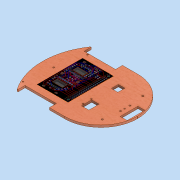
# Autodesk Inventor part: Version Raspberry Pi 3 en adelante
Saved by Autodesk Inventor 2022 (Build 260153000, 153)
## iProperties
Created: 2021-09-27
Part Number: Version Raspberry Pi 3 en adelante
Material: Madera (nogal)
Document SubType Name: Modeling
Designer: Julio R
Density: 0.55 g/cm^3
Appearance: Nogal - Natural pulido
Author: Julio R
Autodesk Inventor part; units mm, degrees
ref_plane "YZ Plane" through (0, 0, 0) normal (1, 0, 0) x (0, 1, 0)
ref_plane "XZ Plane" through (0, 0, 0) normal (0, 1, 0) x (-1, 0, 0)
ref_plane "XY Plane" through (0, 0, 0) normal (0, 0, 1) x (1, 0, 0)
sketch "Boceto2" plane through (0, 0, 0) normal (0, 1, 0) x (-1, 0, 0)
  line L0 (-78.5, 29.7) -> (-78.5, -49.3)
  line L1 (-75.5, -52.3) -> (-25.5, -52.3)
  line L2 (-22.5, -49.3) -> (-22.5, 29.7)
  line L3 (-25.5, 32.7) -> (-75.5, 32.7)
  circle A0 centre (-75, -28.8) radius 1.25
  line L4 (0, 6.809) -> (0, -6.809)
  line L5 (10.65, 0) -> (-10.65, 0) construction
  circle A1 centre (-26, -28.8) radius 1.25
  circle A2 centre (-75, 29.2) radius 1.25
  circle A3 centre (-26, 29.2) radius 1.25
  line L6 (7.5, -42.3) -> (-7, -42.3)
  line L7 (-7, -42.3) -> (-7, -25)
  line L8 (-7, -25) -> (7.5, -25)
  line L9 (7.5, -25) -> (7.5, -42.3)
  arc A4 (9.0958, -33.5419) -> (9.0958, -25.0441) centre (9, -29.293) ccw
  line L10 (9.0958, -33.5419) -> (7.5, -42.3)
  line L11 (9.0958, -25.0441) -> (7.5, -25.0441)
  arc A5 (9.5, -30.443) -> (9.5, -28.143) centre (9.5, -29.293) ccw
  line L12 (9.5, -30.443) -> (7.5, -30.443)
  line L13 (7.5, -30.443) -> (7.5, -28.143)
  line L14 (7.5, -28.143) -> (9.5, -28.143)
  line L15 (9.5, -28.143) -> (9.5, -30.443)
  arc A6 (-9.0958, -25.0441) -> (-9.0958, -33.5419) centre (-9, -29.293) ccw
  line L16 (-9.0958, -33.5419) -> (-7, -42.3)
  line L17 (-9.0958, -25.0441) -> (-7.5, -25.0441)
  arc A7 (-9.5, -28.143) -> (-9.5, -30.443) centre (-9.5, -29.293) ccw
  line L18 (-9.5, -30.443) -> (-7.5, -30.443)
  line L19 (-7.5, -30.443) -> (-7.5, -28.143)
  line L20 (-7.5, -28.143) -> (-9.5, -28.143)
  line L21 (-9.5, -28.143) -> (-9.5, -30.443)
  line L22 (7.5, 42.3) -> (-7, 42.3)
  line L23 (-7, 42.3) -> (-7, 25)
  line L24 (-7, 25) -> (7.5, 25)
  line L25 (7.5, 25) -> (7.5, 42.3)
  arc A8 (9.0958, 25.0441) -> (9.0958, 33.5419) centre (9, 29.293) ccw
  line L26 (9.0958, 33.5419) -> (7.5, 42.3)
  line L27 (9.0958, 25.0441) -> (7.5, 25.0441)
  arc A9 (9.5, 28.143) -> (9.5, 30.443) centre (9.5, 29.293) ccw
  line L28 (9.5, 30.443) -> (7.5, 30.443)
  line L29 (7.5, 30.443) -> (7.5, 28.143)
  line L30 (7.5, 28.143) -> (9.5, 28.143)
  line L31 (9.5, 28.143) -> (9.5, 30.443)
  line L32 (-9.0958, 25.0441) -> (-7.5, 25.0441)
  line L33 (-7.5, 28.143) -> (-9.5, 28.143)
  line L34 (-7.5, 30.443) -> (-7.5, 28.143)
  line L35 (-9.5, 28.143) -> (-9.5, 30.443)
  line L36 (-9.5, 30.443) -> (-7.5, 30.443)
  arc A10 (-9.5, 30.443) -> (-9.5, 28.143) centre (-9.5, 29.293) ccw
  line L37 (-9.0958, 33.5419) -> (-7, 42.3)
  arc A11 (-9.0958, 33.5419) -> (-9.0958, 25.0441) centre (-9, 29.293) ccw
  line L38 (10.3604, -4.25) -> (-9.8396, -4.25)
  line L39 (-9.8396, -4.25) -> (-9.8396, 4.25)
  line L40 (-9.8396, 4.25) -> (10.3604, 4.25)
  line L41 (10.3604, 4.25) -> (10.3604, -4.25)
  line L42 (35.3604, -42.3) -> (-82.3941, -42.3)
  line L43 (-82.3941, -42.3) -> (-82.3941, 42.3)
  line L44 (-82.3941, 42.3) -> (35.3604, 42.3)
  line L45 (35.3604, 42.3) -> (35.3604, -42.3)
  line L46 (-84.1886, -12.75) -> (-94.1886, -12.75)
  line L47 (-94.1886, -12.75) -> (-94.1886, 12.75)
  line L48 (-94.1886, 12.75) -> (-84.1886, 12.75)
  line L49 (-84.1886, 12.75) -> (-84.1886, -12.75)
  line L50 (22.5, 52.3) -> (-22.5, 52.3)
  line L51 (-22.5, 52.3) -> (-22.5, 42.3)
  line L52 (-22.5, 42.3) -> (22.5, 42.3)
  line L53 (22.5, 42.3) -> (22.5, 52.3)
  line L54 (22.5, -52.3) -> (-22.5, -52.3)
  line L55 (-22.5, -52.3) -> (-22.5, -42.3)
  line L56 (-22.5, -42.3) -> (22.5, -42.3)
  line L57 (22.5, -42.3) -> (22.5, -52.3)
  line L58 (22.5, 52.3) -> (23.5693, 52.3)
  line L59 (-22.5, 52.3) -> (-44.8693, 52.3)
  line L60 (22.5, -52.3) -> (23.5693, -52.3)
  line L61 (-22.5, -52.3) -> (-44.8693, -52.3)
  circle A12 centre (-77.6976, 5.7579) radius 1.15
  circle A13 centre (-77.6976, -7.7041) radius 1.15
  arc A14 (23.5693, -52.3) -> (23.5693, 52.3) centre (-52.609, 0) ccw
  line L62 (7.5, -18) -> (-7, -18)
  line L63 (-7, -18) -> (-7, -11.2)
  line L64 (-7, -11.2) -> (7.5, -11.2)
  line L65 (7.5, -11.2) -> (7.5, -18)
  line L66 (7.5, 11.5) -> (-7, 11.5)
  line L67 (-7, 11.5) -> (-7, 18.3)
  line L68 (-7, 18.3) -> (7.5, 18.3)
  line L69 (7.5, 18.3) -> (7.5, 11.5)
  circle A15 centre (24.1703, -0.4774) radius 1
  circle A16 centre (11.6311, 0) radius 1
  circle A17 centre (-11.1103, 0) radius 1
  arc A18 (-22.5, 29.7) -> (-25.5, 32.7) centre (-25.5, 29.7) ccw
  arc A19 (-25.5, -52.3) -> (-22.5, -49.3) centre (-25.5, -49.3) ccw
  arc A20 (-78.5, -49.3) -> (-75.5, -52.3) centre (-75.5, -49.3) ccw
  arc A21 (-75.5, 32.7) -> (-78.5, 29.7) centre (-75.5, 29.7) ccw
  line L70 (-22.5, 26.17) -> (-29.0456, 26.17)
  line L71 (-29.0456, 26.17) -> (-29.0456, -25.7515)
  line L72 (-29.0456, -25.7515) -> (-22.5, -25.7515)
  line L73 (-22.5, -25.7515) -> (-22.5, 26.17)
  line L74 (34.1703, -37.9774) -> (14.1703, -37.9774) construction
  line L75 (14.1703, -37.9774) -> (14.1703, 37.0226) construction
  line L76 (14.1703, 37.0226) -> (34.1703, 37.0226) construction
  line L77 (34.1703, 37.0226) -> (34.1703, -37.9774) construction
  circle A22 centre (28.6937, 39.0367) radius 1
  circle A23 centre (15.9449, -40.5329) radius 1
  circle A24 centre (-41.703, 23.4086) radius 1
  circle A25 centre (-41.703, 11.5) radius 1
  line L78 (-9.7082, -10.0259) -> (10.2918, -10.0259)
  line L79 (10.2918, -10.0259) -> (10.2918, 9.9741)
  line L80 (10.2918, 9.9741) -> (-9.7082, 9.9741)
  line L81 (-9.7082, 9.9741) -> (-9.7082, -10.0259)
  circle A26 centre (-77.6976, -0.0259) radius 1
  line L82 (23.5693, -52.3) -> (-96.2378, -52.3)
  line L83 (-96.2378, -52.3) -> (-96.2378, 52.3)
  line L84 (-96.2378, 52.3) -> (23.5693, 52.3)
  line L85 (55.9366, 25.0441) -> (55.9366, 25)
  line L86 (-22.5, -31.0038) -> (-78.5, -31.0038)
  line L87 (-78.5, -31.0038) -> (-78.5, -52.3)
  line L88 (-78.5, -52.3) -> (-22.5, -52.3)
  line L89 (-22.5, -52.3) -> (-22.5, -31.0038)
  line L90 (10.2918, -10.0259) -> (12.8978, -10.0259)
  line L91 (12.8978, -10.0259) -> (12.8978, -3.1001)
  line L92 (12.8978, -3.1001) -> (10.2918, -3.1001)
  line L93 (10.2918, -3.1001) -> (10.2918, -10.0259)
  line L94 (10.2918, 9.9741) -> (12.8978, 9.9741)
  line L95 (12.8978, 9.9741) -> (12.8978, 3.9285)
  line L96 (12.8978, 3.9285) -> (10.2918, 3.9285)
  line L97 (10.2918, 3.9285) -> (10.2918, 9.9741)
  line L98 (-9.7082, -10.0259) -> (-11.8268, -10.0259)
  line L99 (-11.8268, -10.0259) -> (-11.8268, -3.1001)
  line L100 (-11.8268, -3.1001) -> (-9.7082, -3.1001)
  line L101 (-9.7082, -3.1001) -> (-9.7082, -10.0259)
  line L102 (-9.7082, 9.9741) -> (-11.8268, 9.9741)
  line L103 (-11.8268, 9.9741) -> (-11.8268, 3.9285)
  line L104 (-11.8268, 3.9285) -> (-9.7082, 3.9285)
  line L105 (-9.7082, 3.9285) -> (-9.7082, 9.9741)
  point P0 (0, 0)
  point P1 (-22.5, -52.3)
  point P2 (-22.5, 32.7)
  point P3 (-22.5, -9.8)
  point P4 (0, 0)
  point P5 (13.25, -29.293)
  point P6 (10.65, -29.293)
  point P7 (-13.25, -29.293)
  point P8 (-10.65, -29.293)
  point P9 (13.25, 29.293)
  point P10 (10.65, 29.293)
  point P11 (-10.65, 29.293)
  point P12 (-13.25, 29.293)
  point P13 (-16, 0)
  point P14 (10.3604, 0)
  point P15 (-84.1886, 0)
  point P16 (-7.5, 36.9)
  point P17 (-7.5, 39.2)
  point P18 (-7.5, -39.2)
  point P19 (-7.5, -36.9)
  point P20 (7.5, -28.143)
  point P21 (7.5, -30.443)
  point P22 (-7, -42.3)
  point P23 (7.5, -42.3)
  point P24 (7.5, 42.3)
  point P25 (-7, 42.3)
  point P26 (0, 52.3)
  point P27 (-22.5, -42.3)
  point P28 (22.5, -42.3)
  point P29 (22.5, 42.3)
  point P30 (-22.5, -25.7515)
  point P31 (-7, 42.3)
  point P32 (-9.7082, 4.25)
  point P33 (10.2918, 4.25)
  point P34 (10.2918, -4.25)
  point P35 (-9.7082, -4.25)
  point P36 (-9.8396, -3.1001)
  point P37 (-9.8396, 3.9285)
  point P38 (10.3604, 3.9285)
  point P39 (10.3604, -3.1001)
  dimension "d52" = 85
  dimension "d53" = 56
  dimension "d56" = 3.5
  dimension "d60" = 49
  dimension "d63" = 58
  dimension "d78" = 14.5
  dimension "d79" = 17.3
  dimension "d81" = 1.5
  dimension "d82" = 4.25
  dimension "d83" = 1.15
  dimension "d84" = 2.3
  dimension "d86" = 2
  dimension "d88" = 7.5
  dimension "d92" = 20.2
  dimension "d93" = 8.5
  dimension "d94" = 10
  dimension "d95" = 25.5
  dimension "d108" = 10
  dimension "d113" = 45
  dimension "d114" = 13.462
  dimension "d116" = 2.3
  dimension "d119" = 2.3
  dimension "d127" = 25
  dimension "d134" = 42.3
  dimension "d135" = 1.5958
  dimension "d136" = 14.5
  dimension "d137" = 6.8
  dimension "d138" = 14.5
  dimension "d139" = 6.8
  dimension "d140" = 2
  dimension "d144" = 2
  dimension "d145" = 2
  dimension "d156" = 23
  dimension "d157" = 7
  dimension "d159" = 3
  dimension "d160" = 1.2707
  dimension "d161" = 1.2707
  dimension "d164" = 75
  dimension "d165" = 20
  dimension "d166" = 37.5
  dimension "d168" = 2
  dimension "d169" = 2
  dimension "d170" = 2
  dimension "d171" = 2
  dimension "d177" = 6.5457
  dimension "d179" = 51.9215
  dimension "d181" = 11.9086
  dimension "d182" = 20
  dimension "d183" = 20
  dimension "d387" = 2
  dimension "d421" = 1.7946
  dimension "d465" = 6.491
  dimension "d477" = 9.6
  dimension "d479" = 6.53
  dimension "d480" = 3.5
  dimension "d484" = 22.5
  constraints: 212 end point, 41 symmetric about line, 36 parallel, 28 point on circle, 27 centre point, 20 horizontal, 18 perpendicular, 18 point on line, 8 tangent, 6 midpoint, 6 vertical alignment, 4 collinear, 4 horizontal alignment, 3 coincident, 3 equal radius, 2 vertical, 12 other
  measures "d52" distance of point (-22.5, 32.7) point (-22.5, -52.3)
  measures "d53" distance of point (-22.5, -52.3) L87.end
  measures "d56" horizontal distance of A0.centre L87.end
  measures "d60" distance of A0.centre A1.centre
  measures "d63" distance of A0.centre A2.centre
  measures "d78" distance of L7.end L8.end
  measures "d79" distance of L6.end L7.end
  measures "d81" distance from line of L9 A4.centre
  measures "d82" radius of A4
  measures "d83" radius of A5
  measures "d84" distance between parallel lines of L14 L12
  measures "d86" distance from line of L13 A5.centre
  measures "d88" distance from line of point (0, 0) L9
  measures "d92" distance of L39.end L40.end
  measures "d93" distance of L38.end L39.end
  measures "d94" distance between parallel lines of L47 L49
  measures "d95" distance between parallel lines of L48 L46
  measures "d108" distance of L51.end L50.end
  measures "d113" distance between parallel lines of L51 L53
  measures "d114" distance of A13.centre A12.centre
  measures "d116" diameter of A12
  measures "d119" diameter of A13
  measures "d127" distance between parallel lines of L45 L41
  measures "d134" distance from line of point (0, 0) L42
  measures "d135" distance from line of L9 L11.start
  measures "d136" distance of L63.end L64.end
  measures "d137" distance of L62.end L63.end
  measures "d138" distance of L67.end L68.end
  measures "d139" distance of L66.end L67.end
  measures "d140" diameter of A15
  measures "d144" diameter of A16
  measures "d145" diameter of A17
  measures "d156" diameter of L66 L5
  measures "d157" distance between parallel lines of L8 L62
  measures "d159" radius of A18
  measures "d160" distance from line of L41 A16.centre
  measures "d161" distance from line of L39 A17.centre
  measures "d164" distance between parallel lines of L76 L74
  measures "d165" distance between parallel lines of L75 L77
  measures "d166" distance from line of A15.centre L76
  measures "d168" diameter of A22
  measures "d169" diameter of A23
  measures "d170" diameter of A24
  measures "d171" diameter of A25
  measures "d177" distance between parallel lines of L73 L71
  measures "d179" distance between parallel lines of L70 L72
  measures "d181" distance of A25.centre A24.centre
  measures "d182" distance of L80.end L79.end
  measures "d183" distance of L79.end L78.end
  measures "d387" diameter of A26
  measures "d421" distance between parallel lines of L49 L43
  measures "d465" distance from line of L49 A26.centre
  measures "d477" distance between parallel lines of L44 L3
  measures "d479" distance between parallel lines of L3 L70
  measures "d480" distance from line of L3 A2.centre
  measures "d484" distance from line of L73 point (0, 0)
extrude "Extrusión4" add sketch "Boceto2" along normal blind 3 contours A21 L3 A18 L2 L70 L71 L72 L86 L0 A13 A26 A12 | L0 A12 A26 A13 L42 L43 L44 L23 L24 L25 L27 A8 L26 A14 L45 L10 A4 L11 L9 L8 L7 L2 A18 L3 A21 | L2 L42 L0 L86 | L2 A19 L1 A20 L0 L42 | L0 L87 L82 L83 L84 L59 L51 L44 L43 L42 | L55 L61 A19 | L7 L8 L9 L6 | A20 L82 L87 | L9 L12 A5 L14 L11 A4 L10 | L57 L42 A14 L60 | L22 L25 L24 L23 | L45 A14 | L26 A8 L27 L25 L30 A9 L28 | L58 A14 L44 L53 | L40 L39 L104 L103 L102 L81 | L79 L94 L95 L96 L41 L40 | L38 L41 L92 L91 L90 L79 | L81 L98 L99 L100 L39 L38
fillet "Empalme7" radius 52 2 edges at (96.2378, 1.5, -52.3) (96.2378, 1.5, 52.3)
sketch "Boceto3" plane through (0, 3, 0) normal (0, 1, 0) x (1, 0, 0)
  line L0 (20.8865, 32.3) -> (20.8865, -32.7)
  line L1 (20.8865, -32.7) -> (-14.1135, -32.7)
  line L2 (-14.1135, -32.7) -> (-14.1135, 32.3)
  line L3 (20.8865, 32.3) -> (-14.1135, 32.3)
  circle A0 centre (26, 28.8) radius 1.25 projected
  circle A1 centre (26, -29.2) radius 1.25 projected
  circle A2 centre (41.703, -11.5) radius 1 projected
  circle A3 centre (41.703, -23.4086) radius 1 projected
  circle A4 centre (-28.6937, -39.0367) radius 1 projected
  line L4 (29.0456, 25.7515) -> (29.0456, -26.17) projected
  line L5 (29.0456, -26.17) -> (22.5, -26.17) projected
  line L6 (22.5, -26.17) -> (22.5, 25.7515) projected
  line L7 (22.5, 25.7515) -> (29.0456, 25.7515) projected
  circle A5 centre (-15.9449, 40.5329) radius 1 projected
  circle A6 centre (-24.1703, 0.4774) radius 1 projected
  line L8 (22.5, 52.3) -> (22.5, 42.3) projected
  line L9 (22.5, 42.3) -> (-22.5, 42.3) projected
  line L10 (-22.5, 42.3) -> (-22.5, 52.3) projected
  arc A7 (-23.5693, 52.3) -> (-23.5693, -52.3) centre (52.609, 0) ccw projected
  line L11 (-22.5, -52.3) -> (-22.5, -42.3) projected
  line L12 (-22.5, -42.3) -> (22.5, -42.3) projected
  line L13 (22.5, -42.3) -> (22.5, -52.3) projected
  line L14 (-7.5, 11.2) -> (-7.5, 18) projected
  line L15 (-7.5, 18) -> (7, 18) projected
  line L16 (7, 18) -> (7, 11.2) projected
  line L17 (7, 11.2) -> (-7.5, 11.2) projected
  circle A8 centre (75, -29.2) radius 1.25 projected
  arc A9 (-9.5, 30.443) -> (-9.5, 28.143) centre (-9.5, 29.293) ccw projected
  line L18 (-9.5, 30.443) -> (-7.5, 30.443) projected
  line L19 (-7.5, 30.443) -> (-7.5, 28.143) projected
  line L20 (-7.5, 28.143) -> (-9.5, 28.143) projected
  line L21 (84.1886, -12.75) -> (84.1886, 12.75) projected
  line L22 (84.1886, 12.75) -> (94.1886, 12.75) projected
  line L23 (94.1886, 12.75) -> (94.1886, -12.75) projected
  line L24 (94.1886, -12.75) -> (84.1886, -12.75) projected
  circle A10 centre (77.6976, 7.7041) radius 1.15 projected
  line L25 (-7.5, -30.443) -> (-9.5, -30.443) projected
  arc A11 (-9.5, -28.143) -> (-9.5, -30.443) centre (-9.5, -29.293) ccw projected
  line L26 (-9.5, -28.143) -> (-7.5, -28.143) projected
  line L27 (-7.5, -28.143) -> (-7.5, -30.443) projected
  circle A12 centre (26, 28.8) radius 1.25 projected
  line L28 (-7.5, -18.3) -> (-7.5, -11.5) projected
  line L29 (-7.5, -11.5) -> (7, -11.5) projected
  line L30 (7, -11.5) -> (7, -18.3) projected
  line L31 (7, -18.3) -> (-7.5, -18.3) projected
  circle A13 centre (11.1103, 0) radius 1 projected
  circle A14 centre (26, -29.2) radius 1.25 projected
  line L32 (7.5, 30.443) -> (9.5, 30.443) projected
  arc A15 (9.5, 28.143) -> (9.5, 30.443) centre (9.5, 29.293) ccw projected
  line L33 (9.5, 28.143) -> (7.5, 28.143) projected
  line L34 (7.5, 28.143) -> (7.5, 30.443) projected
  circle A16 centre (77.6976, -5.7579) radius 1.15 projected
  arc A17 (9.5, -30.443) -> (9.5, -28.143) centre (9.5, -29.293) ccw projected
  line L35 (9.5, -30.443) -> (7.5, -30.443) projected
  line L36 (7.5, -30.443) -> (7.5, -28.143) projected
  line L37 (7.5, -28.143) -> (9.5, -28.143) projected
  circle A18 centre (75, 28.8) radius 1.25 projected
  line L38 (-10.3604, -4.25) -> (-10.3604, 4.25) projected
  line L39 (9.8396, 4.25) -> (9.8396, -4.25) projected
  circle A19 centre (-11.6311, 0) radius 1 projected
  line L40 (-15.606, -33.2472) -> (-15.606, 32.7528) construction
  line L41 (-15.606, 32.7528) -> (21.4726, 32.7528) construction
  line L42 (21.4726, 32.7528) -> (21.4726, -33.2472) construction
  line L43 (21.4726, -33.2472) -> (-15.606, -33.2472) construction
  line L44 (-9.0297, -25.5314) -> (9.3868, -25.5314)
  line L45 (9.3868, -25.5314) -> (9.3868, -22.2663)
  line L46 (9.3868, -22.2663) -> (-9.0297, -22.2663)
  line L47 (-9.0297, -22.2663) -> (-9.0297, -25.5314)
  line L48 (-9.0297, 20.6397) -> (7.7218, 20.6397)
  line L49 (7.7218, 20.6397) -> (7.7218, 24.3886)
  line L50 (7.7218, 24.3886) -> (-9.0297, 24.3886)
  line L51 (-9.0297, 24.3886) -> (-9.0297, 20.6397)
  line L52 (22.5, -26.17) -> (22.5, 25.7515) projected
  line L53 (9.3868, -32.0744) -> (22.5, -32.0744)
  line L54 (22.5, -32.0744) -> (22.5, -12.5)
  line L55 (22.5, -12.5) -> (9.3868, -12.5)
  line L56 (9.3868, -12.5) -> (9.3868, -32.0744)
  line L57 (-13.8057, -19.8238) -> (-9.4895, -19.8238)
  line L58 (-9.4895, -19.8238) -> (-9.4895, -4.6772)
  line L59 (-9.4895, -4.6772) -> (-13.8057, -4.6772)
  line L60 (-13.8057, -4.6772) -> (-13.8057, -19.8238)
  line L61 (-13.3666, 8.9365) -> (-9.4895, 8.9365)
  line L62 (-9.4895, 8.9365) -> (-9.4895, 15.1891)
  line L63 (-9.4895, 15.1891) -> (-13.3666, 15.1891)
  line L64 (-13.3666, 15.1891) -> (-13.3666, 8.9365)
  line L65 (-9.4895, -9.55) -> (10.9255, -9.55)
  line L66 (10.9255, -9.55) -> (10.9255, -6.55)
  line L67 (10.9255, -6.55) -> (-9.4895, -6.55)
  line L68 (-9.4895, -6.55) -> (-9.4895, -9.55)
  line L69 (-9.4895, 5.75) -> (10.9255, 5.75)
  line L70 (10.9255, 5.75) -> (10.9255, 8.75)
  line L71 (10.9255, 8.75) -> (-9.4895, 8.75)
  line L72 (-9.4895, 8.75) -> (-9.4895, 5.75)
  line L73 (9.3868, -12.5) -> (7.3247, -12.5)
  line L74 (7.3247, -12.5) -> (7.3247, -21.1057)
  line L75 (7.3247, -21.1057) -> (9.3868, -21.1057)
  line L76 (9.3868, -21.1057) -> (9.3868, -12.5)
  line L77 (52.609, 15.5566) -> (43.1767, 15.5566)
  line L78 (43.1767, 15.5566) -> (43.1767, 25.7515)
  line L79 (43.1767, 25.7515) -> (52.609, 25.7515)
  line L80 (52.609, 25.7515) -> (52.609, 15.5566)
  line L81 (53.8576, -27.3152) -> (43.1767, -27.3152)
  line L82 (43.1767, -27.3152) -> (43.1767, -12.5)
  line L83 (43.1767, -12.5) -> (53.8576, -12.5)
  line L84 (53.8576, -12.5) -> (53.8576, -27.3152)
  line L85 (94.1886, 12.75) -> (97.5693, 12.75)
  line L86 (94.1886, -12.75) -> (84.1886, -12.75) projected
  line L87 (94.1886, -12.75) -> (71.8357, -12.75)
  line L88 (-22.5, 52.3) -> (-23.5693, 52.3) projected
  line L89 (-23.5693, -52.3) -> (-22.5, -52.3) projected
  line L90 (22.5, -52.3) -> (44.2378, -52.3) projected
  line L91 (96.2378, -0.3) -> (96.2378, 0.3) projected
  line L92 (44.2378, 52.3) -> (22.5, 52.3) projected
  line L93 (9.8396, -4.25) -> (9.7082, -4.25) projected
  line L94 (9.7082, -4.25) -> (9.7082, -9.9741) projected
  line L95 (9.7082, -9.9741) -> (-10.2918, -9.9741) projected
  line L96 (-10.2918, -9.9741) -> (-10.2918, -4.25) projected
  line L97 (-10.2918, -4.25) -> (-10.3604, -4.25) projected
  line L98 (-10.3604, 4.25) -> (-10.2918, 4.25) projected
  line L99 (-10.2918, 4.25) -> (-10.2918, 10.0259) projected
  line L100 (-10.2918, 10.0259) -> (9.7082, 10.0259) projected
  line L101 (9.7082, 10.0259) -> (9.7082, 4.25) projected
  line L102 (9.7082, 4.25) -> (9.8396, 4.25) projected
  arc A20 (44.2378, -52.3) -> (96.2378, -0.3) centre (44.2378, -0.3) ccw projected
  arc A21 (96.2378, 0.3) -> (44.2378, 52.3) centre (44.2378, 0.3) ccw projected
  point P0 (0, 0)
  dimension "d184" = 35
  dimension "d185" = 65
  dimension "d186" = 3.5
  dimension "d187" = 3.5
  dimension "d188" = 6.8
  dimension "d189" = 6.6135
  dimension "d193" = 2.257
  dimension "d194" = 1.857
  dimension "d196" = 14.5
  dimension "d197" = 6.8
  dimension "d198" = 14.5
  dimension "d200" = 6.6135
  dimension "d202" = 14.4
  dimension "d203" = 13.8865
  dimension "d204" = 43.9
  dimension "d205" = 31.247
  dimension "d206" = 28.45
  dimension "d207" = 2
  dimension "d209" = 13.3865
  dimension "d210" = 13.3865
  dimension "d211" = 15
  dimension "d212" = 13.3865
  dimension "d213" = 28.3865
  dimension "d331" = 66
  dimension "d377" = 3
  dimension "d378" = 3
  constraints: 92 end point, 20 parallel, 12 horizontal, 11 perpendicular, 7 point on line, 3 vertical, 1 collinear, 2 other
  measures "d184" distance of L0.start L2.end
  measures "d185" distance of L1.end L2.end
  measures "d186" distance from line of L3 A0.centre
  measures "d187" distance from line of L1 A1.centre
  measures "d188" distance between parallel lines of L17 L15
  measures "d189" distance between parallel lines of L2 L14
  measures "d193" distance between parallel lines of L1 L35
  measures "d194" distance between parallel lines of L3 L32
  measures "d196" distance between parallel lines of L14 L16
  measures "d197" distance between parallel lines of L31 L29
  measures "d198" distance between parallel lines of L28 L30
  measures "d200" distance between parallel lines of L2 L28
  measures "d202" vertical distance of L0.end L30.end
  measures "d203" horizontal distance of L0.end L30.end
  measures "d204" vertical distance of L0.end L16.end
  measures "d205" horizontal distance of L0.end L38.start
  measures "d206" vertical distance of L0.end L38.start
  measures "d207" distance from line of A15.centre L34
  measures "d209" horizontal distance of L0.start L32.start
  measures "d210" distance between parallel lines of L0 L36
  measures "d211" distance between parallel lines of L36 L27
  measures "d212" distance from line of L0.start L34
  measures "d213" distance between parallel lines of L0 L19
  measures "d331" distance of L40.start L40.end
  measures "d377" distance between parallel lines of L69 L71
  measures "d378" distance between parallel lines of L65 L67
extrude "Extrusión13" cut sketch "Boceto3" against normal blind 3 contours L67 L94 L65 L58 | L67 L66 L65 L94 | L101 L69 L72 L71 | L71 L70 L69 L101 | L77 L78 L79 L80 | L81 L82 L83 L84
sketch "Boceto4" plane through (0, 3, 0) normal (0, 1, 0) x (1, 0, 0)
  line L0 (-15.3527, -32.737) -> (-15.3527, 32.8228) construction
  line L1 (-15.3527, 32.8228) -> (29.504, 32.8228) construction
  line L2 (29.504, 32.8228) -> (29.504, -32.737) construction
  line L3 (29.504, -32.737) -> (-15.3527, -32.737) construction
  point P0 (0, 0)
  constraints: 2 other
extrude "Extrusión15" cut sketch "Boceto2" along normal blind 3 contours L40 L39 L104 L103 L102 L81 | L79 L94 L95 L96 L41 L40 | L38 L41 L92 L91 L90 L79 | L81 L98 L99 L100 L39 L38
